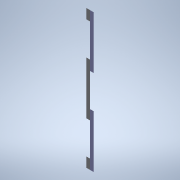
# Autodesk Inventor part: PinturaDetectores
Saved by Autodesk Inventor 2021.2 (Build 252289000, 289)
## iProperties
Created: 2026-10-05
Part Number: PinturaDetectores
Material: Generic
Document SubType Name: Modeling
Designer: nelso
Density: 1 g/cm^3
Appearance: Default
Author: nelso
Autodesk Inventor part; units mm, degrees
ref_plane "YZ Plane" through (0, 0, 0) normal (1, 0, 0) x (0, 1, 0)
ref_plane "XZ Plane" through (0, 0, 0) normal (0, 1, 0) x (-1, 0, 0)
ref_plane "XY Plane" through (0, 0, 0) normal (0, 0, 1) x (1, 0, 0)
sketch "Sketch1" plane through (0, 0, 0) normal (0, 1, 0) x (-1, 0, 0)
  line L0 (30, 565) -> (-30, 565)
  line L1 (-30, 565) -> (-30, -565)
  line L2 (-30, -565) -> (30, -565)
  line L3 (30, -565) -> (30, 565)
  line L4 (30, 565) -> (-30, -565) construction
  line L5 (-30, 565) -> (30, -565) construction
  line L6 (30, -565) -> (0, -565)
  line L7 (0, -565) -> (0, -485)
  line L8 (0, -485) -> (30, -485)
  line L9 (30, -485) -> (30, -565)
  line L10 (-30, -565) -> (0, -565)
  line L11 (0, -565) -> (0, -135)
  line L12 (0, -135) -> (-30, -135)
  line L13 (-30, -135) -> (-30, -565)
  line L14 (30, -135) -> (30, -215)
  line L15 (30, -215) -> (0, -215)
  line L16 (0, -215) -> (0, 215)
  line L17 (0, 215) -> (30, 215)
  line L18 (30, 215) -> (30, -215)
  line L19 (0, 215) -> (0, 135)
  line L20 (0, 135) -> (-30, 135)
  line L21 (-30, 135) -> (-30, 565)
  line L22 (-30, 565) -> (0, 565)
  line L23 (0, 565) -> (0, 135)
  line L24 (30, 565) -> (0, 565)
  line L25 (0, 565) -> (0, 485)
  line L26 (0, 485) -> (30, 485)
  line L27 (30, 485) -> (30, 565)
  point P0 (0, 0)
  dimension "d0" = 60
  dimension "d1" = 1130
  dimension "d2" = 80
  dimension "d3" = 430
  dimension "d4" = 80
  dimension "d5" = 430
  dimension "d6" = 80
  dimension "d7" = 430
  dimension "d8" = 80
  constraints: 56 end point, 12 parallel, 6 horizontal, 6 perpendicular, 5 point on line, 2 midpoint
  measures "d0" distance of L2.end L1.end
  measures "d1" distance of L1.end L0.end
  measures "d2" distance of L6.end L7.end
  measures "d3" distance of L11.end L10.end
  measures "d4" distance of L14.start L14.end
  measures "d5" distance of L15.end L16.end
  measures "d6" distance of L16.end L19.end
  measures "d7" distance of L20.end L0.end
  measures "d8" distance of L25.end L24.end
extrude "Extrusion1" add sketch "Sketch1" along normal blind 0.01 contours L3 L26 L23 L0 | L3 L15 L11 L16 L17 | L3 L2 L7 L8
extrude "Extrusion2" add sketch "Sketch1" along normal blind 0.01 separate body contours L23 L16 L20 L1 L0 | L12 L11 L7 L2 L1
body "Solid1"
body "Solid2"
